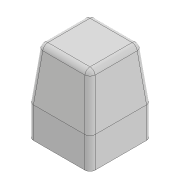
# Autodesk Inventor part: raida-
Saved by Autodesk Inventor 2020 (Build 240168000, 168)
## iProperties
Created: 2020-04-18
Part Number: raida-
Material: 一般
Document SubType Name: Modeling
Designer: highs
Density: 1 g/cm^3
Appearance: 既定
Author: highs
Autodesk Inventor part; units mm, degrees
ref_plane "YZ Plane" through (0, 0, 0) normal (1, 0, 0) x (0, 1, 0)
ref_plane "XZ Plane" through (0, 0, 0) normal (0, 1, 0) x (-1, 0, 0)
ref_plane "XY Plane" through (0, 0, 0) normal (0, 0, 1) x (1, 0, 0)
sketch "スケッチ1" plane through (0, 0, 0) normal (0, 1, 0) x (-1, 0, 0)
  line L0 (0, 0) -> (60, 0)
  line L1 (60, 0) -> (60, -60)
  line L2 (60, -60) -> (0, -60)
  line L3 (0, -60) -> (0, 0)
  dimension "d0" = 60
  dimension "d1" = 60
  constraints: 8 end point, 2 parallel, 1 horizontal, 1 perpendicular
  measures "d0" distance of L0.start L0.end
  measures "d1" distance of L2.end L0.start
extrude "押し出し1" add sketch "スケッチ1" along normal blind 80
chamfer "面取り1" distance 5 distance2 50 1 edges at (0, 80, -30) measured on face at (-20, 80, -40)
chamfer "面取り2" distance 5 distance2 50 1 edges at (-60, 80, -30) measured on face at (-23.3333, 80, -40)
chamfer "面取り3" distance 5 distance2 50 1 edges at (-30, 80, -60) measured on face at (-21.6667, 80, -40)
chamfer "面取り4" distance 5 distance2 50 1 edges at (-30, 80, 0) measured on face at (-21.6667, 80, -18.3333)
fillet "フィレット1" radius 5 12 edges at (0, 15, -60) (-60, 15, -60) (-60, 15, 0) (0, 15, 0) (-57.5, 55, -2.5) (-57.5, 55, -57.5) (-55, 80, -30) (-30, 80, -5) (-5, 80, -30) (-30, 80, -55) (-2.5, 55, -2.5) (-2.5, 55, -57.5)
sketch "スケッチ2" plane through (0, 0, 0) normal (0, -1, 0) x (1, 0, 0)
  line L0 (-60, -55) -> (-60, -5) projected
  line L1 (-60, -30) -> (0, -30) construction
  line L2 (0, -5) -> (0, -55) projected
  line L3 (-55, -19.95) -> (-5, -19.95)
  line L4 (-5, -19.95) -> (-5, -40.05)
  line L5 (-5, -40.05) -> (-55, -40.05)
  line L6 (-55, -40.05) -> (-55, -19.95)
  line L7 (-55, -19.95) -> (-5, -40.05) construction
  line L8 (-5, -19.95) -> (-55, -40.05) construction
  point P0 (0, 0)
  point P1 (-30, -30)
  dimension "d17" = 50
  dimension "d18" = 20.1
  constraints: 14 end point, 5 midpoint, 2 parallel, 1 horizontal, 1 perpendicular
  measures "d17" distance of L3.start L3.end
  measures "d18" distance of L3.end L4.end
extrude "押し出し2" cut sketch "スケッチ2" against normal blind 1
